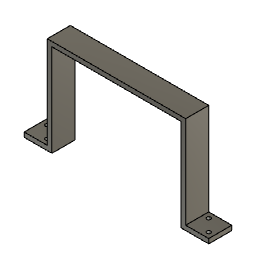
Ceinture alim SAE (Autodesk Fusion 360 design; units mm, degrees)
Autodesk Fusion 360 part; units mm, degrees
sketch "Esquisse1" plane through (0, 0, 0) normal (0, 0, 1) x (1, 0, 0)
  line L0 (0, 0) -> (140, 0)
  line L1 (140, 0) -> (140, -150)
  line L2 (140, -150) -> (0, -150)
  line L3 (0, -150) -> (0, 0)
  dimension "d1" = 140
  dimension "d2" = 150
  constraint horizontal L0
  constraint vertical L1
  constraint horizontal L2
  constraint vertical L3
  constraint coincident L0.start L3.end
  measures "d1" distance of L0.start L0.end
  measures "d2" distance of L0.start L2.end
extrude "Extrusion1" add sketch "Esquisse1" along normal blind 100 makes body 1
sketch "Esquisse2" plane through (0, 0, 100) normal (0, 0, 1) x (-1, 0, 0)
  line L0 (0, 150) -> (-140, 150)
  line L1 (-140, 150) -> (-140, 0)
  line L2 (-140, 0) -> (0, 0)
  line L3 (0, 0) -> (0, 150)
  line L4 (0, 50) -> (-140, 50)
  line L5 (-140, 50) -> (-140, 75)
  line L6 (-140, 75) -> (0, 75)
  line L7 (0, 75) -> (0, 50)
  constraint horizontal L4
  constraint vertical L5
  constraint horizontal L6
  constraint vertical L7
  constraint midpoint L1 L5.end
  constraint coincident L3 L4.start
extrude "Extrusion2" add sketch "Esquisse2" along normal blind 5 separate body contours L1 L3 L4 L5 L6 L7 makes body 2
sketch "Esquisse3" plane through (140, 0, 0) normal (1, 0, 0) x (0, 1, 0)
  line L0 (-150, 0) -> (0, 0)
  line L1 (0, 0) -> (0, 100)
  line L2 (0, 100) -> (-150, 100)
  line L3 (-150, 100) -> (-150, 0)
  line L4 (-75, 105) -> (-50, 105)
  line L5 (-50, 105) -> (-50, 0)
  line L6 (-50, 0) -> (-75, 0)
  line L7 (-75, 0) -> (-75, 105)
  constraint horizontal L4
  constraint vertical L5
  constraint horizontal L6
  constraint vertical L7
  constraint coincident L0 L5.end
extrude "Extrusion3" add sketch "Esquisse3" along normal blind 5 separate body contours L0 L2 L5 L6 L7 | L2 L4 L5 L7 makes body 3
sketch "Esquisse4" plane through (0, 0, 0) normal (-1, 0, 0) x (0, -1, 0)
  line L0 (50, 100) -> (75, 100)
  line L1 (75, 100) -> (75, 105)
  line L2 (75, 105) -> (50, 105)
  line L3 (50, 105) -> (50, 100)
  line L4 (50, 105) -> (75, 105)
  line L5 (75, 105) -> (75, 0)
  line L6 (75, 0) -> (50, 0)
  line L7 (50, 0) -> (50, 105)
  dimension "d9" = 25
  constraint horizontal L4
  constraint vertical L5
  constraint horizontal L6
  constraint vertical L7
  constraint coincident L2.end L3.start
  measures "d9" distance of L2.end L1.end
extrude "Extrusion4" add sketch "Esquisse4" along normal blind 5 separate body makes body 4
sketch "Esquisse6" plane through (0, 0, 0) normal (0, 0, 1) x (1, 0, 0)
  line L0 (-5, -75) -> (-30, -75)
  line L1 (-30, -75) -> (-30, -50)
  line L2 (-30, -50) -> (-5, -50)
  line L3 (-5, -50) -> (-5, -75)
  line L4 (145, -50) -> (170, -50)
  line L5 (170, -50) -> (170, -75)
  line L6 (170, -75) -> (145, -75)
  line L7 (145, -75) -> (145, -50)
  circle A0 centre (-24, -56) radius 2.125
  circle A1 centre (-11, -69) radius 2.125
  circle A2 centre (151, -56) radius 2.125
  circle A3 centre (164, -69) radius 2.125
  dimension "d12" = 4.25
  dimension "d13" = 4.25
  dimension "d14" = 6
  dimension "d15" = 6
  dimension "d16" = 6
  dimension "d17" = 6
  dimension "d18" = 4.25
  dimension "d19" = 4.25
  dimension "d20" = 6
  dimension "d21" = 6
  dimension "d22" = 6
  dimension "d23" = 6
  constraint horizontal L0
  constraint vertical L1
  constraint horizontal L2
  constraint vertical L3
  constraint horizontal L4
  constraint vertical L5
  constraint horizontal L6
  constraint vertical L7
  measures "d12" diameter of A0
  measures "d13" diameter of A1
  measures "d14" distance of L1 A0.centre
  measures "d15" distance of L2 A0.centre
  measures "d16" distance of L3 A1.centre
  measures "d17" distance of L0 A1.centre
  measures "d18" diameter of A2
  measures "d19" diameter of A3
  measures "d20" distance of L5 A3.centre
  measures "d21" distance of L6 A3.centre
  measures "d22" distance of L4 A2.centre
  measures "d23" distance of L7 A2.centre
extrude "Extrusion5" add sketch "Esquisse6" along normal blind 5 bodies 3 4
combine "Combiner1" operation add target body 2 tool bodies 3 4
hidden bodies 1
named bodies: "Alim", "Ceinture"
